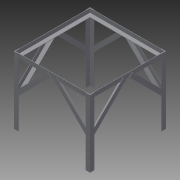
# Autodesk Inventor part: Single_Burner_Stand
Saved by Autodesk Inventor 2014 (Build 180170000, 170)
## iProperties
Created: 2016-08-25
Part Number: Single_Burner_Stand
Material: Generic
Document SubType Name: Modeling
Designer: jmw3
Density: 1 g/cm^3
Appearance: Default
Author: jmw3
Autodesk Inventor part; units mm, degrees
ref_plane "YZ Plane" through (0, 0, 0) normal (1, 0, 0) x (0, 1, 0)
ref_plane "XZ Plane" through (0, 0, 0) normal (0, 1, 0) x (-1, 0, 0)
ref_plane "XY Plane" through (0, 0, 0) normal (0, 0, 1) x (1, 0, 0)
sketch "Sketch1" plane through (0, 0, 0) normal (0, 1, 0) x (-1, 0, 0)
  line L0 (0, -471.17) -> (0, 471.17) projected
  line L1 (471.17, 0) -> (-471.17, 0) projected
  line L2 (-333.375, 333.375) -> (333.375, 333.375)
  line L3 (333.375, 333.375) -> (333.375, -333.375)
  line L4 (333.375, -333.375) -> (-333.375, -333.375)
  line L5 (-333.375, -333.375) -> (-333.375, 333.375)
  line L6 (-298.45, 298.45) -> (298.45, 298.45)
  line L7 (298.45, 298.45) -> (298.45, -298.45)
  line L8 (298.45, -298.45) -> (-298.45, -298.45)
  line L9 (-298.45, -298.45) -> (-298.45, 298.45)
  line L10 (-336.55, 336.55) -> (336.55, 336.55)
  line L11 (336.55, 336.55) -> (336.55, -336.55)
  line L12 (336.55, -336.55) -> (-336.55, -336.55)
  line L13 (-336.55, -336.55) -> (-336.55, 336.55)
  point P0 (0, 0)
  dimension "d0" = 666.75
  dimension "d1" = 666.75
  dimension "d4" = 3.175
  dimension "d5" = 3.175
  dimension "d50" = 38.1
  dimension "d51" = 38.1
  constraints: 24 end point, 6 parallel, 3 horizontal, 3 perpendicular, 6 other
  measures "d0" distance between parallel lines of L3 L5
  measures "d1" distance between parallel lines of L4 L2
  measures "d4" distance between parallel lines of L5 L13
  measures "d5" distance between parallel lines of L4 L12
  measures "d50" distance between parallel lines of L13 L9
  measures "d51" distance between parallel lines of L10 L6
extrude "Extrusion1" add sketch "Sketch1" against normal blind 3.175 contours L12 L13 L1 L5 L4 L0 | L0 L4 L3 L1 L11 L12 | L4 L5 L1 L9 L8 L0 | L0 L8 L7 L1 L3 L4 | L1 L3 L2 L0 L10 L11 | L13 L10 L0 L2 L5 L1 | L1 L7 L6 L0 L2 L3 | L5 L2 L0 L6 L9 L1
extrude "Extrusion2" add sketch "Sketch1" along normal blind 34.925 contours L12 L13 L1 L5 L4 L0 | L0 L4 L3 L1 L11 L12 | L1 L3 L2 L0 L10 L11 | L13 L10 L0 L2 L5 L1
sketch "Sketch2" plane through (0, 34.925, 0) normal (0, 1, 0) x (1, 0, 0)
  line L0 (336.55, -336.55) -> (336.55, 336.55) projected
  line L1 (336.55, 336.55) -> (-336.55, 336.55) projected
  line L2 (301.625, 336.55) -> (336.55, 336.55)
  line L3 (339.725, 339.725) -> (301.625, 339.725)
  line L4 (301.625, 339.725) -> (301.625, 336.55)
  line L5 (339.725, 339.725) -> (339.725, 301.625)
  line L6 (339.725, 301.625) -> (336.55, 301.625)
  line L7 (336.55, 301.625) -> (336.55, 336.55)
  point P0 (0, 0)
  dimension "d10" = 3.175
  dimension "d15" = 3.175
  dimension "d52" = 38.1
  dimension "d53" = 38.1
  constraints: 12 end point, 2 parallel, 1 collinear, 1 horizontal, 1 point on line
  measures "d10" distance between parallel lines of L2 L3
  measures "d15" distance between parallel lines of L0 L5
  measures "d52" distance between parallel lines of L5 L4
  measures "d53" distance between parallel lines of L3 L6
extrude "Extrusion3" add sketch "Sketch2" against normal blind 601.6625
sketch "Sketch4" plane through (336.55, -3.175, 336.55) normal (1, 0, 0) x (0, 0, -1)
  line L0 (673.1, 0) -> (0, 0) projected
  line L1 (377.7476, 24.6957) -> (350.8068, -2.2451)
  line L2 (350.8068, -2.2451) -> (638.175, -289.6133)
  line L3 (638.175, -289.6133) -> (638.175, -235.7317)
  line L4 (638.175, -235.7317) -> (377.7476, 24.6957)
  line L5 (638.175, 38.1) -> (638.175, -563.5625) projected
  line L6 (676.275, -563.5625) -> (638.175, -563.5625) projected
  line L7 (353.0519, 0) -> (638.175, -285.1231)
  line L8 (353.0519, 0) -> (350.8068, -2.2451)
  line L9 (350.8068, -2.2451) -> (638.175, -289.6133)
  line L10 (638.175, -289.6133) -> (638.175, -285.1231)
  line L11 (638.175, -285.1231) -> (353.0519, 0)
  point P0 (336.55, 3.175)
  point P1 (676.275, -339.725)
  dimension "d23" = 38.1
  dimension "d28" = 3.175
  dimension "d47" = 45
  dimension "d49" = 406.4
  constraints: 18 end point, 4 perpendicular, 3 parallel, 3 point on line, 2 collinear, 1 other
  measures "d23" distance of L1.start L1.end
  measures "d28" distance between parallel lines of L2 L7
  measures "d47" angle of L5 L4
  measures "d49" distance from line of L2.end L1
extrude "Extrusion5" add sketch "Sketch4" against normal blind 34.925 contours L7 L3 L2 L1
extrude "Extrusion6" add sketch "Sketch4" along normal blind 3.175 contours L4 L3 L7 L0 | L0 L1 L4 | L7 L3 L2 L1
sketch "Sketch5" plane through (339.725, 34.925, -339.725) normal (0, 0, -1) x (-1, 0, 0)
  line L0 (38.1, 0) -> (38.1, -601.6625) projected
  line L1 (676.275, -38.1) -> (38.1, -38.1) projected
  line L2 (676.275, 0) -> (676.275, -38.1) projected
  line L3 (38.1, 0) -> (676.275, 0) projected
  line L4 (38.1, -327.7133) -> (325.4682, -40.3451)
  line L5 (325.4682, -40.3451) -> (298.5274, -13.4043)
  line L6 (298.5274, -13.4043) -> (38.1, -273.8317)
  line L7 (38.1, -273.8317) -> (38.1, -327.7133)
  line L8 (323.2231, -38.1) -> (38.1, -323.2231)
  line L9 (38.1, 0) -> (38.1, -38.1) projected
  point P0 (0, -381)
  point P1 (339.725, -34.925)
  dimension "d33" = 38.1
  dimension "d35" = 3.175
  dimension "d45" = 45
  dimension "d48" = 406.4
  constraints: 10 end point, 5 point on line, 3 perpendicular, 1 parallel
  measures "d33" distance of L4.end L5.end
  measures "d35" distance between parallel lines of L4 L8
  measures "d45" angle of L0 L6
  measures "d48" distance from line of L5 L4.start
extrude "Extrusion7" add sketch "Sketch5" against normal blind 3.175 contours L6 L1 L8 L0 | L6 L5 L1 | L8 L5 L4 L0
extrude "Extrusion8" add sketch "Sketch5" against normal blind 38.1 contours L8 L5 L4 L0
mirror "Mirror1" about plane through (0, 0, 0) normal (0, 0, 1) of "Extrusion8", "Extrusion7", "Extrusion6", "Extrusion5", "Extrusion3"
mirror "Mirror2" about plane through (0, 0, 0) normal (1, 0, 0) of "Extrusion8", "Extrusion7", "Extrusion6", "Extrusion5", "Extrusion3", "Mirror1"
body "Solid1"
